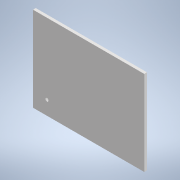
# Autodesk Inventor part: BasePlate
Saved by Autodesk Inventor 2020 (Build 240168000, 168)
## iProperties
Created: 2019-06-17
Part Number: BasePlate
Material: Generic
Document SubType Name: Modeling
Designer: amirt
Density: 1 g/cm^3
Appearance: Default
Author: amirt
Autodesk Inventor part; units mm, degrees
ref_plane "YZ Plane" through (0, 0, 0) normal (1, 0, 0) x (0, 1, 0)
ref_plane "XZ Plane" through (0, 0, 0) normal (0, 1, 0) x (-1, 0, 0)
ref_plane "XY Plane" through (0, 0, 0) normal (0, 0, 1) x (1, 0, 0)
sketch "Sketch1" plane through (0, 0, 0) normal (0, 0, 1) x (1, 0, 0)
  line L0 (12.7, 0) -> (12.7, 12.7)
  line L1 (12.7, 12.7) -> (0, 12.7)
  circle A0 centre (-76, -52) radius 1.4224 projected
  line L2 (-88.7, -52) -> (-88.7, -64.7)
  line L3 (-88.7, -64.7) -> (-76, -64.7)
  line L4 (-88.7, -64.7) -> (12.7, -64.7)
  line L5 (12.7, -64.7) -> (12.7, 12.7)
  line L6 (12.7, 12.7) -> (-88.7, 12.7)
  line L7 (-88.7, 12.7) -> (-88.7, -64.7)
  point P0 (0, 0)
  dimension "d0" = 12.7
  dimension "d1" = 12.7
  dimension "d2" = 12.7
  dimension "d3" = 12.7
  constraints: 16 end point, 2 parallel, 1 horizontal, 1 perpendicular
  measures "d0" distance of L1.end L0.end
  measures "d1" distance of L0.end L0.start
  measures "d2" distance of L3.end L2.end
  measures "d3" distance of L2.end L2.start
extrude "Extrusion1" add sketch "Sketch1" along normal blind 2.54 contours L5 L4 L3 L2 L7 L6 L1 L0 | A0
body "Solid1"
